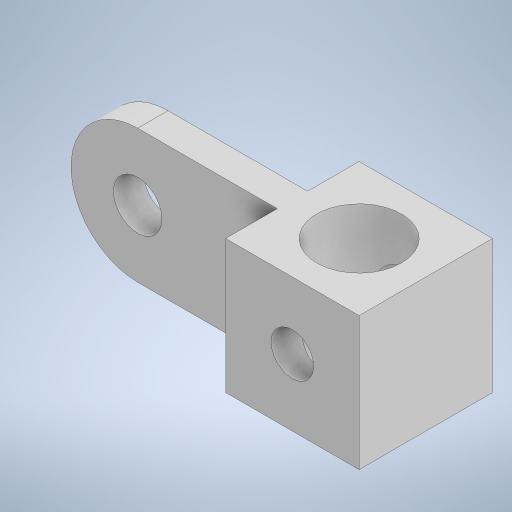
# Autodesk Inventor part: 17_UnionA
Saved by Autodesk Inventor 2024.2 (Build 282272000, 272)
## iProperties
Created: 2024-04-27
Part Number: 17_UnionA
Material: Genérico
Document SubType Name: Modeling
Designer: Cosmic Dinodog
Density: 1 g/cm^3
Appearance: Valor por defecto
Author: Cosmic Dinodog
Autodesk Inventor part; units mm, degrees
ref_plane "YZ Plane" through (0, 0, 0) normal (1, 0, 0) x (0, 1, 0)
ref_plane "XZ Plane" through (0, 0, 0) normal (0, 1, 0) x (-1, 0, 0)
ref_plane "XY Plane" through (0, 0, 0) normal (0, 0, 1) x (1, 0, 0)
sketch "Boceto1" plane through (0, 0, 0) normal (0, 1, 0) x (-1, 0, 0)
  line L0 (11, 11) -> (-11, 11)
  line L1 (-11, 11) -> (-11, -11)
  line L2 (-11, -11) -> (11, -11)
  line L3 (11, -11) -> (11, 11)
  line L4 (11, -11) -> (-11, 11) construction
  line L5 (-11, -11) -> (11, 11) construction
  circle A0 centre (0, 0) radius 7 construction
  point P0 (0, 0)
  point P1 (0, 0)
  dimension "d0" = 22
  dimension "d1" = 22
  dimension "d2" = 22
  dimension "d3" = 14
  constraints: 12 end point, 2 midpoint, 2 perpendicular, 1 centre point, 1 coincident, 1 horizontal
  measures "d0" distance of L0.start L0.end
  measures "d1" distance of L0.end L1.end
  measures "d2" distance of L1.end L2.end
  measures "d3" diameter of A0
extrude "Extrusión1" add sketch "Boceto1" along normal blind 22
sketch "Boceto2" plane through (0, 0, 0) normal (0, 0, 1) x (1, 0, 0)
  line L0 (0, 0) -> (0, 11) construction
  line L1 (0, 11) -> (-34, 11) construction
  circle A0 centre (-34, 11) radius 4
  arc A1 (-34, 22) -> (-34, 0) centre (-34, 11) ccw
  line L2 (-11, 0) -> (11, 0) projected
  line L3 (11, 0) -> (11, 22) projected
  line L4 (-11, 22) -> (11, 22) projected
  line L5 (-11, 0) -> (-11, 22) projected
  line L6 (-34, 0) -> (-11, 0)
  line L7 (-34, 22) -> (-11, 22)
  line L8 (-11, 22) -> (-11, 0)
  dimension "d6" = 11
  dimension "d8" = 34
  dimension "d9" = 8
  dimension "d10" = 22
  constraints: 10 end point, 2 centre point, 2 coincident, 2 point on circle, 2 tangent, 1 collinear, 1 horizontal, 1 vertical
  measures "d6" distance of L0.start L0.end
  measures "d8" distance of L0.end L1.end
  measures "d9" diameter of A0
  measures "d10" diameter of A1
extrude "Extrusión2" add sketch "Boceto2" along normal mid plane 5 contours L7 L5 L6 A1
sketch "Boceto3" plane through (-11, 0, 11) normal (0, 0, 1) x (1, 0, 0)
  line L0 (0, 0) -> (0, 11) construction
  line L1 (0, 0) -> (0, 22) projected
  line L2 (0, 11) -> (11, 11) construction
  circle A0 centre (11, 11) radius 3.5
  line L3 (0, 0) -> (22, 0) projected
  point P0 (11, 0)
  point P1 (11, 0)
  dimension "d14" = 7
  dimension "d15" = 11
  constraints: 4 end point, 2 midpoint, 1 centre point, 1 coincident, 1 perpendicular
  measures "d14" diameter of A0
  measures "d15" distance of point (11, 0) L2.end
extrude "Extrusión3" cut sketch "Boceto3" against normal through all
sketch "Boceto4" plane through (0, 22, 0) normal (0, 1, 0) x (1, 0, 0)
  circle A0 centre (0, 0) radius 7
  dimension "d18" = 14
  constraints: 1 centre point, 1 coincident
  measures "d18" diameter of A0
extrude "Extrusión4" cut sketch "Boceto4" against normal through all
